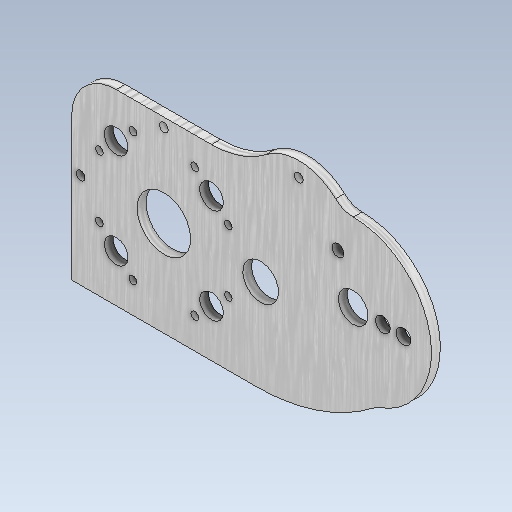
# Autodesk Inventor part: 中間フレーム
Saved by Autodesk Inventor 2020.4 (Build 244396000, 396)
## iProperties
Created: 2021-04-23
Part Number: 中間フレーム
Material: アルミニウム 7075
Document SubType Name: Modeling
Designer: happy
Density: 2.81 g/cm^3
Appearance: サテン - ブラシ仕上げ 重厚
Mass: 54.4848 g
Surface Area: 150.293 cm^2
Volume: 19.3896 cm^3
Author: happy
Autodesk Inventor part; units mm, degrees
ref_plane "YZ Plane" through (0, 0, 0) normal (1, 0, 0) x (0, 1, 0)
ref_plane "XZ Plane" through (0, 0, 0) normal (0, 1, 0) x (-1, 0, 0)
ref_plane "XY Plane" through (0, 0, 0) normal (0, 0, 1) x (1, 0, 0)
sketch "スケッチ1" plane through (0, 0, 0) normal (0, 0, 1) x (1, 0, 0)
  line L0 (65.0196, -14.5) -> (65.0196, 33.6804)
  circle A0 centre (80.0196, 33.6804) radius 15 construction
  line L1 (80.0196, 48.6804) -> (112.2, 48.6804)
  circle A1 centre (112.2, 33.6804) radius 15 construction
  line L2 (127.2, -14.5) -> (65.0196, -14.5)
  circle A2 centre (80.0196, 33.6804) radius 3.05 construction
  circle A3 centre (112.2, 33.6804) radius 3.05 construction
  circle A4 centre (112.2, 1.5) radius 3.05 construction
  circle A5 centre (80.0196, 1.5) radius 3.05 construction
  circle A6 centre (96.1098, 17.5902) radius 2.85 construction
  circle A7 centre (128.7687, 16.8502) radius 5.7 construction
  circle A8 centre (160, 25) radius 21.5 construction
  circle A9 centre (128.7687, 16.8502) radius 28.5 construction
  circle A10 centre (128.7687, 16.8502) radius 29.4672 construction
  circle A11 centre (160, 25) radius 25.8772 construction
  circle A12 centre (80.0196, 33.6804) radius 4
  circle A13 centre (112.2, 33.6804) radius 4
  circle A14 centre (80.0196, 1.5) radius 4
  circle A15 centre (112.2, 1.5) radius 4
  arc A16 (112.2, 48.6804) -> (130.0806, 54.5913) centre (112.2, 78.6804) ccw
  arc A17 (153.3164, 53.0826) -> (160, 50.3812) centre (160, 60) ccw
  arc A18 (153.3164, 53.0826) -> (130.0806, 54.5913) centre (140.809, 40.1379) ccw
  circle A19 centre (96.1098, 17.5902) radius 9.025
  circle A20 centre (128.7687, 16.8502) radius 6.025
  circle A21 centre (160, 25) radius 5
  arc A22 (168.6809, 1.1495) -> (160, 50.3812) centre (160, 25) ccw
  arc A23 (168.6809, 1.1495) -> (165.807, -0.5048) centre (171.9707, -7.8892) ccw
  circle A24 centre (171.9707, -7.8892) radius 8.6188 construction
  arc A25 (127.2, -14.5) -> (165.807, -0.5048) centre (127.2, 45.748) ccw
  circle A26 centre (160, 60) radius 8.6188 construction
  circle A27 centre (154.8697, 39.0954) radius 3 construction
  circle A28 centre (154.8697, 39.0954) radius 2
  arc A29 (157.2213, 29.1568) -> (99.1742, 26.079) centre (128.7687, 16.8502) ccw construction
  arc A30 (98.7866, 8.9713) -> (159.6067, 20.0155) centre (128.7687, 16.8502) ccw construction
  arc A31 (80.0196, 48.6804) -> (65.0196, 33.6804) centre (80.0196, 33.6804) ccw
  circle A32 centre (68.0196, 17.5902) radius 1.5
  circle A33 centre (96.1098, 45.6804) radius 1.5
  circle A34 centre (74.3628, 28.0235) radius 1.3
  circle A35 centre (85.6765, 39.3372) radius 1.3
  circle A36 centre (106.5431, 39.3372) radius 1.3
  circle A37 centre (117.8569, 28.0235) radius 1.3
  circle A38 centre (117.8569, 7.1569) radius 1.3
  circle A39 centre (106.5431, -4.1569) radius 1.3
  circle A40 centre (85.6765, -4.1569) radius 1.3
  circle A41 centre (74.3628, 7.1569) radius 1.3
  line L3 (74.3628, 28.0235) -> (85.6765, 39.3372) construction
  line L4 (65.0196, -14.5) -> (65.0196, 33.6804)
  circle A42 centre (80.0196, 33.6804) radius 15 construction
  line L5 (80.0196, 48.6804) -> (112.2, 48.6804)
  circle A43 centre (112.2, 33.6804) radius 15 construction
  line L6 (127.2, -14.5) -> (65.0196, -14.5)
  circle A44 centre (80.0196, 33.6804) radius 3.05 construction
  circle A45 centre (112.2, 33.6804) radius 3.05 construction
  circle A46 centre (112.2, 1.5) radius 3.05 construction
  circle A47 centre (80.0196, 1.5) radius 3.05 construction
  circle A48 centre (96.1098, 17.5902) radius 2.85 construction
  circle A49 centre (128.7687, 16.8502) radius 5.7 construction
  circle A50 centre (160, 25) radius 21.5 construction
  circle A51 centre (128.7687, 16.8502) radius 28.5 construction
  circle A52 centre (128.7687, 16.8502) radius 29.4672 construction
  circle A53 centre (160, 25) radius 25.8772 construction
  circle A54 centre (80.0196, 33.6804) radius 6
  circle A55 centre (112.2, 33.6804) radius 6
  circle A56 centre (80.0196, 1.5) radius 6
  circle A57 centre (112.2, 1.5) radius 6
  arc A58 (112.2, 48.6804) -> (130.5847, 54.9738) centre (112.2, 78.6804) ccw
  arc A59 (154.0473, 53.767) -> (160, 51.3812) centre (160, 60) ccw
  arc A60 (154.0473, 53.767) -> (130.5847, 54.9738) centre (141.6155, 40.7498) ccw
  circle A61 centre (96.1098, 17.5902) radius 9.025
  circle A62 centre (128.7687, 16.8502) radius 6.025
  circle A63 centre (160, 25) radius 2
  arc A64 (169.0229, 0.2098) -> (160, 51.3812) centre (160, 25) ccw
  arc A65 (169.0229, 0.2098) -> (166.7152, -1.0582) centre (171.9707, -7.8892) ccw
  circle A66 centre (171.9707, -7.8892) radius 8.6188 construction
  arc A67 (127.2, -14.5) -> (166.7152, -1.0582) centre (127.2, 50.3027) ccw
  circle A68 centre (160, 60) radius 8.6188 construction
  circle A69 centre (154.8697, 39.0954) radius 3 construction
  circle A70 centre (154.8697, 39.0954) radius 2
  arc A71 (158.348, 26.1273) -> (99.1742, 26.079) centre (128.7687, 16.8502) ccw construction
  arc A72 (98.7866, 8.9713) -> (159.1094, 23.2092) centre (128.7687, 16.8502) ccw construction
  arc A73 (80.0196, 48.6804) -> (65.0196, 33.6804) centre (80.0196, 33.6804) ccw
  circle A74 centre (141.6155, 53.7498) radius 5 construction
  circle A75 centre (141.6155, 53.7498) radius 4
  circle A76 centre (141.6155, 53.7498) radius 1.5
  point P0 (0, 0)
  point P1 (0, 0)
  point P2 (96.1924, 17.5902)
  point P3 (80.1022, 1.5)
  point P4 (112.2826, 1.5)
  point P5 (112.2826, 33.6804)
  point P6 (80.1962, 33.857)
  point P7 (160, 60)
  point P8 (0, 0)
  point P9 (96.1924, 17.5902)
  point P10 (80.1022, 1.5)
  point P11 (112.2826, 1.5)
  point P12 (112.2826, 33.6804)
  point P13 (80.1022, 33.6804)
  point P14 (160, 60)
  point P15 (148.0694, -11.0476)
  point P16 (129.8149, 10.9168)
  point P17 (127.7224, 22.7837)
  point P18 (97.677, 8.7023)
  point P19 (94.5426, 26.4781)
  dimension "d0" = 8
  dimension "d1" = 30
  dimension "d2" = 18.05
  dimension "d3" = 12.05
  dimension "d4" = 10
  dimension "d5" = 1
  dimension "d6" = 18
  dimension "d7" = 4
  dimension "d8" = 31
  dimension "d9" = 32.2772
  dimension "d10" = 60.248
  dimension "d13" = 3
  dimension "d14" = 3
  dimension "d15" = 2.6
  dimension "d16" = 16
  dimension "d25" = 12
  dimension "d26" = 30
  dimension "d27" = 18.05
  dimension "d28" = 12.05
  dimension "d29" = 4
  dimension "d30" = 0
  dimension "d31" = 18
  dimension "d32" = 4
  dimension "d33" = 31
  dimension "d34" = 64.8027
  dimension "d35" = 10
  dimension "d36" = 8
  dimension "d37" = 3
  constraints: 73 centre point, 45 point on circle, 20 coincident, 19 tangent, 15 equal radius, 14 end point, 6 concentric, 4 vertical alignment, 2 horizontal, 1 midpoint, 1 point on line, 1 vertical, 37 other
  measures "d0" diameter of A13
  measures "d1" radius of A16
  measures "d2" diameter of A19
  measures "d3" diameter of A20
  measures "d4" diameter of A21
  measures "d5" radial gap between concentric circles of A24 A23
  measures "d6" radius of A18
  measures "d7" diameter of A28
  measures "d8" radius of A29
  measures "d9" distance of A20.centre A21.centre
  measures "d10" radius of A25
  measures "d13" diameter of A32
  measures "d14" diameter of A33
  measures "d15" diameter of A34
  measures "d16" distance of L3.end L3.start
  measures "d25" diameter of A55
  measures "d26" radius of A58
  measures "d27" diameter of A61
  measures "d28" diameter of A62
  measures "d29" diameter of A63
  measures "d30" radial gap between concentric circles of A66 A65
  measures "d31" radius of A60
  measures "d32" diameter of A70
  measures "d33" radius of A71
  measures "d34" radius of A67
  measures "d35" diameter of A74
  measures "d36" diameter of A75
  measures "d37" diameter of A76
extrude "押し出し1" add sketch "スケッチ1" along normal blind 3 contours L0 A31 L1 A16 A18 A17 A22 A23 A25 L2 | A25 A23 A22 A17 A18 A58 A60 A59 A64 A65 A67 | A54 | A55 | A56 | A57 | A75
sketch "スケッチ2" plane through (0, 0, 0) normal (0, 0, -1) x (-1, 0, 0)
  line L0 (-65.0196, -14.5) -> (-127.2, -14.5) projected
  line L1 (-65.0196, 33.6804) -> (-65.0196, -14.5) projected
  arc A0 (-65.0196, 33.6804) -> (-80.0196, 48.6804) centre (-80.0196, 33.6804) ccw projected
  line L2 (-112.2, 48.6804) -> (-80.0196, 48.6804) projected
  circle A1 centre (-74.3628, 7.1569) radius 1.3 projected
  circle A2 centre (-106.5431, -4.1569) radius 1.3 projected
  circle A3 centre (-117.8569, 28.0235) radius 1.3 projected
  circle A4 centre (-74.3628, 28.0235) radius 1.3 projected
  circle A5 centre (-68.0196, 17.5902) radius 1.5 projected
  circle A6 centre (-96.1098, 45.6804) radius 1.5 projected
  circle A7 centre (-154.8697, 39.0954) radius 2 projected
  circle A8 centre (-128.7687, 16.8502) radius 6.025 projected
  circle A9 centre (-96.1098, 17.5902) radius 9.025 projected
  circle A10 centre (-112.2, 1.5) radius 4 projected
  circle A11 centre (-80.0196, 1.5) radius 4 projected
  circle A12 centre (-112.2, 33.6804) radius 4 projected
  circle A13 centre (-85.6765, 39.3372) radius 1.3 projected
  circle A14 centre (-106.5431, 39.3372) radius 1.3 projected
  circle A15 centre (-117.8569, 7.1569) radius 1.3 projected
  circle A16 centre (-85.6765, -4.1569) radius 1.3 projected
  circle A17 centre (-160, 25) radius 5 projected
  circle A18 centre (-80.0196, 33.6804) radius 4 projected
  circle A19 centre (-170, 25) radius 2.5
  circle A20 centre (-177, 25) radius 2.5
  line L3 (-160, 25) -> (-180.4045, 25) construction
  arc A21 (-166.7152, -1.0582) -> (-127.2, -14.5) centre (-127.2, 50.3027) ccw projected
  arc A22 (-130.5847, 54.9738) -> (-154.0473, 53.767) centre (-141.6155, 40.7498) ccw projected
  arc A23 (-160, 51.3812) -> (-154.0473, 53.767) centre (-160, 60) ccw projected
  arc A24 (-160, 51.3812) -> (-169.0229, 0.2098) centre (-160, 25) ccw projected
  arc A25 (-166.7152, -1.0582) -> (-169.0229, 0.2098) centre (-171.9707, -7.8892) ccw projected
  arc A26 (-130.5847, 54.9738) -> (-112.2, 48.6804) centre (-112.2, 78.6804) ccw projected
  point P0 (0, 0)
  dimension "d20" = 10
  dimension "d21" = 7
  dimension "d22" = 5
  constraints: 2 centre point, 2 end point, 2 point on line, 1 equal radius, 1 horizontal
  measures "d20" distance of L3.start A19.centre
  measures "d21" distance of A19.centre A20.centre
  measures "d22" diameter of A19
extrude "押し出し2" cut sketch "スケッチ2" against normal blind 10 contours A19 | A20
